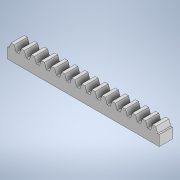
# Autodesk Inventor part: Rack
Saved by Autodesk Inventor 2021 (Build 250183000, 183)
## iProperties
Created: 2025-04-11
Part Number: Rack
Material: Generic
Document SubType Name: Modeling
Designer: Lukas
Density: 1 g/cm^3
Appearance: Default
Author: Lukas
Autodesk Inventor part; units mm, degrees
ref_plane "YZ Plane" through (0, 0, 0) normal (1, 0, 0) x (0, 1, 0)
ref_plane "XZ Plane" through (0, 0, 0) normal (0, 1, 0) x (-1, 0, 0)
ref_plane "XY Plane" through (0, 0, 0) normal (0, 0, 1) x (1, 0, 0)
sketch "Sketch1" plane through (0, 0, 0) normal (0, 0, 1) x (1, 0, 0)
  line L0 (-1.9279, 2) -> (-1.9279, -2)
  line L1 (-1.9279, -2) -> (1.9279, -2)
  line L2 (1.9279, -2) -> (1.9279, 2)
  line L3 (-1.9279, 2) -> (-1.3279, 2)
  line L4 (-1.3279, 2) -> (-0.6, 4)
  line L5 (-0.6, 4) -> (0.6, 4)
  line L6 (0.6, 4) -> (1.3279, 2)
  line L7 (1.3279, 2) -> (1.9279, 2)
  point P0 (0, 0)
  point P1 (0, 4)
  point P2 (0, -2)
  point P3 (-1.9279, 0)
  dimension "d0" = 1.2
  dimension "d1" = 2
  dimension "d2" = 20
  dimension "d3" = 4
  dimension "d4" = 0.6
  constraints: 16 end point, 3 midpoint, 2 equal length, 2 horizontal alignment, 2 perpendicular, 2 vertical alignment, 1 collinear, 1 horizontal, 1 parallel, 1 point on line, 1 vertical
  measures "d0" distance of L4.end L5.end
  measures "d1" distance between parallel lines of L5 L7
  measures "d2" angle of L2 L6
  measures "d3" distance of L1.end L2.end
  measures "d4" distance of L0.start L3.end
extrude "Extrusion1" add sketch "Sketch1" along normal blind 5
pattern_linear "Rectangular Pattern1" count 15 spacing 3.855 along (1, 0, 0)
equation "\"d4\" = 0.5 * d0"
body "Solid1"
